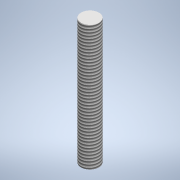
# Autodesk Inventor part: Stift_5mm
Saved by Autodesk Inventor 2021.3 (Build 253353000, 353)
## iProperties
Created: 2021-04-15
Part Number: Stift_5mm
Material: Generic
Document SubType Name: Modeling
Designer: Fabijan_Sven
Density: 1 g/cm^3
Appearance: Default
Author: Fabijan_Sven
Autodesk Inventor part; units mm, degrees
ref_plane "YZ Plane" through (0, 0, 0) normal (1, 0, 0) x (0, 1, 0)
ref_plane "XZ Plane" through (0, 0, 0) normal (0, 1, 0) x (-1, 0, 0)
ref_plane "XY Plane" through (0, 0, 0) normal (0, 0, 1) x (1, 0, 0)
sketch "Sketch1" plane through (0, 0, 0) normal (0, 1, 0) x (-1, 0, 0)
  circle A0 centre (0, 0) radius 2.5
  dimension "d0" = 5
  constraints: 1 centre point, 1 coincident
  measures "d0" diameter of A0
extrude "Extrusion1" add sketch "Sketch1" along normal blind 35
thread "Thread1" size "M5x0.8" class "6g" standard "ISO Metric profile" full length
body "Solid1"
